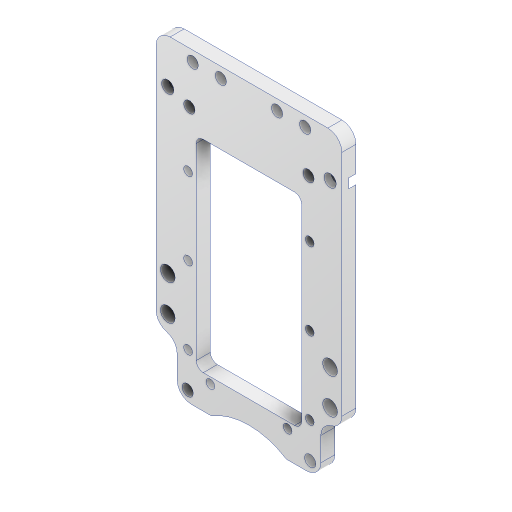
# Autodesk Inventor part: 조인트4고정부
Saved by Autodesk Inventor 2023.2 (Build 272271000, 271)
## iProperties
Created: 2022-01-25
Part Number: 조인트4고정부
Material: 알루미늄 6061
Document SubType Name: Modeling
Designer: BAEK
Density: 2.7 g/cm^3
Appearance: 알루미늄 - 평지
Mass: 26.6199 g
Surface Area: 76.4867 cm^2
Volume: 9.85924 cm^3
Author: BAEK
Autodesk Inventor part; units mm, degrees
ref_plane "YZ Plane" through (0, 0, 0) normal (1, 0, 0) x (0, 1, 0)
ref_plane "XZ Plane" through (0, 0, 0) normal (0, 1, 0) x (-1, 0, 0)
ref_plane "XY Plane" through (0, 0, 0) normal (0, 0, 1) x (1, 0, 0)
sketch "스케치1" plane through (0, 0, 0) normal (0, 0, 1) x (1, 0, 0)
  arc A0 (16.8326, 2) -> (15.3326, 3.5) centre (15.3326, 2) ccw
  line L0 (16.8326, 2) -> (16.8326, 0.5)
  arc A1 (16.8326, 0.5) -> (19.1826, -1.85) centre (19.1826, 0.5) ccw
  line L1 (19.1826, -1.85) -> (21.1826, -1.85)
  arc A2 (22.1826, -2.85) -> (21.1826, -1.85) centre (21.1826, -2.85) ccw
  line L2 (22.1826, -2.85) -> (22.1826, -45.65)
  arc A3 (21.1826, -46.65) -> (22.1826, -45.65) centre (21.1826, -45.65) ccw
  line L3 (21.1826, -46.65) -> (19.1826, -46.65)
  arc A4 (19.1826, -46.65) -> (16.8326, -49) centre (19.1826, -49) ccw
  line L4 (16.8326, -49) -> (16.8326, -51)
  arc A5 (15.8326, -52) -> (16.8326, -51) centre (15.8326, -51) ccw
  line L5 (15.8326, -52) -> (-0.4674, -52)
  arc A6 (-1.4674, -51) -> (-0.4674, -52) centre (-0.4674, -51) ccw
  line L6 (-1.4674, -51) -> (-1.4674, -49)
  arc A7 (-1.4674, -49) -> (-3.8174, -46.65) centre (-3.8174, -49) ccw
  line L7 (-3.8174, -46.65) -> (-5.8174, -46.65)
  arc A8 (-6.8174, -45.65) -> (-5.8174, -46.65) centre (-5.8174, -45.65) ccw
  line L8 (-6.8174, -45.65) -> (-6.8174, -2.85)
  arc A9 (-5.8174, -1.85) -> (-6.8174, -2.85) centre (-5.8174, -2.85) ccw
  line L9 (-5.8174, -1.85) -> (-3.8174, -1.85)
  arc A10 (-3.8174, -1.85) -> (-1.4674, 0.5) centre (-3.8174, 0.5) ccw
  line L10 (-1.4674, 0.5) -> (-1.4674, 2)
  arc A11 (0.0326, 3.5) -> (-1.4674, 2) centre (0.0326, 2) ccw
  circle A12 centre (24.9826, -27.5) radius 1.25
  circle A13 centre (18.6826, -54.8) radius 1.25
  circle A14 centre (-9.6174, -5.5) radius 1.25
  circle A15 centre (-9.6174, -27.5) radius 1.25
  circle A16 centre (-3.3174, -54.8) radius 1.25
  circle A17 centre (24.9826, -49.5) radius 1.25
  circle A18 centre (-9.6174, -49.5) radius 1.25
  circle A19 centre (24.9826, -5.5) radius 1.25
  line L11 (0.0326, 3.5) -> (0.0326, 0.875)
  spline S0 degree 3 poles (0.0326, 0.875) (0.0326, 0.7776) (0.0314, 0.6798) (0.029, 0.5822) (0.0265, 0.4846) (0.0229, 0.3871) (0.0181, 0.29) (0.0132, 0.1929) (0.0072, 0.0961) (0, 0) knots 0 0 0 0 0.333333 0.333333 0.333333 0.666667 0.666667 0.666667 1 1 1 1
  line L12 (15.3652, 0) -> (0, 0)
  spline S1 degree 3 poles (15.3652, 0) (15.3581, 0.0956) (15.352, 0.1921) (15.3472, 0.289) (15.3424, 0.386) (15.3387, 0.4835) (15.3363, 0.5813) (15.3338, 0.679) (15.3326, 0.7771) (15.3326, 0.875) knots 0.000001 0.000001 0.000001 0.000001 0.333333 0.333333 0.333333 0.666667 0.666667 0.666667 1 1 1 1
  line L13 (15.3326, 0.875) -> (15.3326, 3.5)
  line L14 (15.3326, 3.5) -> (0.0326, 3.5)
  circle A20 centre (7.6826, -9.5) radius 5
  line L15 (28.124, 3.5) -> (28.124, -58.5)
  line L16 (-12.7588, 3.5) -> (-12.7588, -58.5)
  line L17 (-12.7588, -58.5) -> (28.124, -58.5)
  line L18 (-12.7588, 3.5) -> (-12.7588, 4.4)
  line L19 (28.124, 4.4) -> (28.124, 3.5)
  line L20 (-12.7588, 4.4) -> (-12.7588, 10)
  line L21 (-12.7588, 10) -> (28.124, 10)
  line L22 (28.124, 10) -> (28.124, 4.4)
  line L23 (7.6826, -52) -> (7.6826, -53)
  line L24 (-6.8174, -24.25) -> (-7.3174, -24.25)
  line L25 (22.1826, -24.25) -> (22.6826, -24.25)
  line L26 (7.6826, 3.5) -> (7.6826, 4.5)
  line L27 (7.6826, 4.5) -> (-5.3174, 4.5)
  line L28 (-7.3174, 2.5) -> (-7.3174, -51)
  line L29 (-5.3174, -53) -> (20.6826, -53)
  line L30 (22.6826, -51) -> (22.6826, 2.5)
  line L31 (20.6826, 4.5) -> (7.6826, 4.5)
  line L32 (-12.7588, -27.5) -> (28.124, -27.5) construction
  line L33 (-3.3174, -54.8) -> (-3.3174, 10) construction
  line L34 (18.6826, -54.8) -> (18.6826, 10) construction
  line L35 (-3.3174, 10) -> (-3.3174, 6.3)
  line L36 (18.6826, 10) -> (18.6826, 6.3)
  circle A21 centre (-3.3174, 6.3) radius 1.25
  circle A22 centre (18.6826, 6.3) radius 1.25
  arc A23 (-7.3174, -51) -> (-5.3174, -53) centre (-5.3174, -51) ccw
  arc A24 (20.6826, -53) -> (22.6826, -51) centre (20.6826, -51) ccw
  arc A25 (22.6826, 2.5) -> (20.6826, 4.5) centre (20.6826, 2.5) ccw
  arc A26 (-5.3174, 4.5) -> (-7.3174, 2.5) centre (-5.3174, 2.5) ccw
  point P0 (0, 0)
  point P1 (-7.3174, 4.5)
  point P2 (-7.3174, -53)
  point P3 (22.6826, -53)
  point P4 (22.6826, 4.5)
  dimension "d4" = 62
  dimension "d9" = 5.6
  dimension "d10" = 1
  dimension "d11" = 0.5
  dimension "d12" = 0.5
  dimension "d13" = 1
  dimension "d14" = 3.7
  dimension "d15" = 3.7
  dimension "d16" = 68.5
  dimension "d18" = 9.4414
  dimension "d19" = 9.4414
  dimension "d22" = 3.7
  dimension "d23" = 3.7
  dimension "d24" = 2.5
  dimension "d25" = 2.5
  dimension "d32" = 2
  dimension "d138" = 2.5
  dimension "d139" = 2.5
  dimension "d140" = 2.5
  dimension "d141" = 2.5
  dimension "d142" = 2.5
  dimension "d143" = 2.5
  dimension "d144" = 2.5
  dimension "d145" = 2.5
  constraints: 74 end point, 32 point on circle, 27 centre point, 12 point on line, 8 tangent, 6 midpoint, 6 perpendicular, 5 horizontal, 5 vertical, 3 equal radius, 2 coincident, 1 parallel, 4 other
  measures "d4" distance of L16.start L16.end
  measures "d9" distance of L18.end L20.end
  measures "d10" distance of L23.start L23.end
  measures "d11" distance of L24.start L24.end
  measures "d12" distance of L25.start L25.end
  measures "d13" distance of L26.start L26.end
  measures "d14" distance from line of L17 L33.start
  measures "d15" distance from line of L17 L34.start
  measures "d16" distance between parallel lines of L17 L21
  measures "d18" distance from line of L16 L33.start
  measures "d19" distance from line of L15 L34.start
  measures "d22" distance of L33.end L35.end
  measures "d23" distance of L34.end L36.end
  measures "d24" diameter of A21
  measures "d25" diameter of A22
  measures "d32" radius of A23
  measures "d138" diameter of A14
  measures "d139" diameter of A15
  measures "d140" diameter of A18
  measures "d141" diameter of A17
  measures "d142" diameter of A12
  measures "d143" diameter of A19
  measures "d144" diameter of A13
  measures "d145" diameter of A16
extrude "돌출2" add sketch "스케치1" along normal blind 4 contours A22 | A21 | L15 L17 L16 L18 L20 L21 L22 L19
sketch "스케치4" plane through (0, 0, 4) normal (0, 0, 1) x (1, 0, 0)
  circle A0 centre (7.6826, -9.5) radius 5
  point P0 (0, 0)
  constraints: 1 centre point
sketch "스케치7" plane through (0, 0, 4) normal (0, 0, 1) x (1, 0, 0)
  line L0 (28.124, 10) -> (-12.7588, 10) projected
  line L1 (-12.7588, 10) -> (28.124, 10)
  line L2 (28.124, 10) -> (28.124, 14)
  line L3 (28.124, 14) -> (-12.7588, 14)
  line L4 (-12.7588, 14) -> (-12.7588, 10)
  line L5 (-12.7588, -58.5) -> (28.124, -58.5) projected
  line L6 (-12.7588, -58.5) -> (28.124, -58.5)
  line L7 (28.124, -58.5) -> (28.124, -62.5)
  line L8 (28.124, -62.5) -> (-12.7588, -62.5)
  line L9 (-12.7588, -62.5) -> (-12.7588, -58.5)
  point P0 (0, 0)
  dimension "d50" = 4
  dimension "d51" = 4
  constraints: 16 end point, 5 perpendicular, 2 horizontal, 1 collinear, 1 point on line
  measures "d50" distance of L0.start L2.end
  measures "d51" distance of L5.end L7.end
extrude "돌출4" add sketch "스케치7" against normal up to surface (4 mm away)
sketch "스케치5" plane through (0, 0, 4) normal (0, 0, 1) x (1, 0, 0)
  line L0 (-12.7588, 14) -> (-12.7588, -62.5) projected
  line L1 (28.124, -62.5) -> (28.124, 14) projected
  circle A0 centre (24.9826, -5.5) radius 1.25 projected
  circle A1 centre (-9.6174, -5.5) radius 1.25 projected
  circle A2 centre (-9.6174, -27.5) radius 1.25 projected
  line L2 (-5.3174, 4.5) -> (20.6826, 4.5) projected
  arc A3 (22.6826, 2.5) -> (20.6826, 4.5) centre (20.6826, 2.5) ccw projected
  line L3 (22.6826, 2.5) -> (22.6826, -51) projected
  arc A4 (20.6826, -53) -> (22.6826, -51) centre (20.6826, -51) ccw projected
  line L4 (20.6826, -53) -> (-5.3174, -53) projected
  arc A5 (-7.3174, -51) -> (-5.3174, -53) centre (-5.3174, -51) ccw projected
  line L5 (-7.3174, -51) -> (-7.3174, 2.5) projected
  arc A6 (-5.3174, 4.5) -> (-7.3174, 2.5) centre (-5.3174, 2.5) ccw projected
  circle A7 centre (-9.6174, -49.5) radius 1.25 projected
  circle A8 centre (-3.3174, -54.8) radius 1.25 projected
  circle A9 centre (24.9826, -49.5) radius 1.25 projected
  circle A10 centre (18.6826, -54.8) radius 1.25 projected
  circle A11 centre (24.9826, -27.5) radius 1.25 projected
  circle A12 centre (-9.7588, -59.5) radius 1.6
  circle A13 centre (25.124, -59.5) radius 1.6
  circle A14 centre (-9.2588, 10.5) radius 1.6
  circle A15 centre (24.624, 10.5) radius 1.6
  line L6 (-12.7588, -62.5) -> (28.124, -62.5) projected
  line L7 (28.124, 14) -> (-12.7588, 14) projected
  point P0 (0, 0)
  dimension "d36" = 3.2
  dimension "d37" = 3.2
  dimension "d38" = 3.2
  dimension "d39" = 3.2
  dimension "d40" = 3
  dimension "d42" = 3.5
  dimension "d44" = 3.5
  dimension "d46" = 3
  dimension "d54" = 3
  dimension "d55" = 3
  dimension "d56" = 3.5
  dimension "d57" = 3.5
  constraints: 4 centre point
  measures "d36" diameter of A12
  measures "d37" diameter of A13
  measures "d38" diameter of A14
  measures "d39" diameter of A15
  measures "d40" distance from line of L0 A12.centre
  measures "d42" distance from line of L0 A14.centre
  measures "d44" distance from line of L1 A15.centre
  measures "d46" distance from line of L1 A13.centre
  measures "d54" distance from line of L6 A12.centre
  measures "d55" distance from line of L6 A13.centre
  measures "d56" distance from line of L7 A14.centre
  measures "d57" distance from line of L7 A15.centre
extrude "돌출3" cut sketch "스케치5" against normal blind 4 contours A12 | A13 | A14 | A15
sketch "스케치8" plane through (0, 0, 4) normal (0, 0, 1) x (1, 0, 0)
  line L0 (-12.7588, 14) -> (28.124, 14) projected
  line L1 (7.6826, 14) -> (7.6826, -136) construction
  circle A0 centre (7.6826, -79.433) radius 20
  line L2 (-12.7588, -62.5) -> (28.124, -62.5) projected
  point P0 (0, 0)
  point P1 (-10.7588, 14)
  point P2 (26.124, 14)
  point P3 (-10.7588, -62.5)
  point P4 (26.124, -62.5)
  point P5 (-2.9604, -62.5)
  point P6 (18.3256, -62.5)
  dimension "d59" = 150
  dimension "d60" = 40
  dimension "d61" = 16.933
  constraints: 2 end point, 1 centre point, 1 midpoint, 1 point on line, 1 vertical
  measures "d59" distance of L1.start L1.end
  measures "d60" diameter of A0
  measures "d61" distance from line of L2 A0.centre
extrude "돌출5" cut sketch "스케치8" against normal up to surface (4 mm away) contours L2 A0 picked at (9.885, -61.852)
sketch "스케치12" plane through (0, 0, 4) normal (0, 0, 1) x (1, 0, 0)
  circle A0 centre (-9.6174, -27.5) radius 1.25 projected
  line L0 (-9.6174, -27.5) -> (-9.6174, -33.6) construction
  line L1 (-9.6174, -33.6) -> (-15.4174, -33.6) construction
  circle A1 centre (-15.4174, -33.6) radius 2.1
  line L2 (-12.7588, 14) -> (-12.7588, -62.5) projected
  line L3 (-15.4174, -33.6) -> (-15.4174, -43.6) construction
  circle A2 centre (-15.4174, -43.6) radius 2.1
  arc A3 (18.3256, -62.5) -> (-2.9604, -62.5) centre (7.6826, -79.433) ccw projected
  line L4 (-15.4174, -33.6) -> (-15.4174, 12.4) construction
  circle A4 centre (-15.4174, 12.4) radius 1.75
  line L5 (28.124, 14) -> (-12.7588, 14) projected
  line L6 (7.6826, 14) -> (7.6826, -59.433) construction
  arc A5 (18.3256, -62.5) -> (-2.9604, -62.5) centre (7.6826, -79.433) ccw projected
  circle A6 centre (30.7826, -33.6) radius 2.1
  line L7 (30.7826, -33.6) -> (30.7826, -43.6) construction
  circle A7 centre (30.7826, -43.6) radius 2.1
  line L8 (30.7826, -33.6) -> (30.7826, 12.4) construction
  circle A8 centre (30.7826, 12.4) radius 1.75
  line L9 (-12.7588, 14) -> (-12.7588, -62.5) projected
  line L10 (-12.7588, 14) -> (-12.7588, 17)
  line L11 (-12.7588, 17) -> (28.124, 17)
  line L12 (28.124, 17) -> (28.124, 14)
  line L13 (28.124, 17) -> (34.124, 17)
  line L14 (34.124, 17) -> (34.124, -48)
  line L15 (34.124, -48) -> (28.124, -48)
  line L16 (28.124, -62.5) -> (28.124, 14) projected
  line L17 (-12.7588, 17) -> (-18.7588, 17)
  line L18 (-18.7588, 17) -> (-18.7588, -48)
  line L19 (-18.7588, -48) -> (-12.7588, -48)
  point P0 (0, 0)
  point P1 (-12.7588, -60.5)
  point P2 (28.124, -60.5)
  dimension "d83" = 6.1
  dimension "d84" = 5.8
  dimension "d85" = 4.2
  dimension "d87" = 10
  dimension "d88" = 4.2
  dimension "d89" = 46
  dimension "d90" = 3
  dimension "d91" = 6
  dimension "d92" = 65
  dimension "d93" = 6
  dimension "d128" = 3.5
  constraints: 32 end point, 6 centre point, 6 coincident, 6 symmetric about line, 6 vertical, 5 perpendicular, 3 point on line, 2 point on circle, 1 midpoint, 1 parallel, 3 other
  measures "d83" distance of L0.start L0.end
  measures "d84" distance of L0.end L1.end
  measures "d85" diameter of A1
  measures "d87" distance of L3.start L3.end
  measures "d88" diameter of A2
  measures "d89" distance of L3.start L4.end
  measures "d90" distance of L2.start L10.end
  measures "d91" distance of L11.end L13.end
  measures "d92" distance of L13.end L14.end
  measures "d93" distance of L10.end L17.end
  measures "d128" diameter of A4
extrude "돌출8" add sketch "스케치12" against normal blind 4 contours L10 L11 L12 L5 | L2 L19 L18 L17 L10 | L12 L13 L14 L15 L16
sketch "스케치13" plane through (0, 0, 4) normal (0, 0, 1) x (1, 0, 0)
  circle A0 centre (-15.4174, 12.4) radius 1.75 projected
  circle A1 centre (-15.4174, -43.6) radius 2.1 projected
  circle A2 centre (-15.4174, -33.6) radius 2.1 projected
  circle A3 centre (30.7826, 12.4) radius 1.75 projected
  circle A4 centre (30.7826, -43.6) radius 2.1 projected
  circle A5 centre (30.7826, -33.6) radius 2.1 projected
  circle A6 centre (24.9826, -27.5) radius 1.25 projected
  circle A7 centre (18.6826, -54.8) radius 1.25 projected
  circle A8 centre (24.9826, -49.5) radius 1.25 projected
  circle A9 centre (-3.3174, -54.8) radius 1.25 projected
  circle A10 centre (-9.6174, -49.5) radius 1.25 projected
  arc A11 (20.6826, -53) -> (22.6826, -51) centre (20.6826, -51) ccw projected
  line L0 (20.6826, -53) -> (-5.3174, -53) projected
  arc A12 (-7.3174, -51) -> (-5.3174, -53) centre (-5.3174, -51) ccw projected
  line L1 (-7.3174, -51) -> (-7.3174, 2.5) projected
  arc A13 (-5.3174, 4.5) -> (-7.3174, 2.5) centre (-5.3174, 2.5) ccw projected
  line L2 (-5.3174, 4.5) -> (20.6826, 4.5) projected
  arc A14 (22.6826, 2.5) -> (20.6826, 4.5) centre (20.6826, 2.5) ccw projected
  line L3 (22.6826, 2.5) -> (22.6826, -51) projected
  circle A15 centre (-9.6174, -27.5) radius 1.25 projected
  circle A16 centre (-9.6174, -5.5) radius 1.25 projected
  circle A17 centre (24.9826, -5.5) radius 1.25 projected
  arc A18 (18.3256, -62.5) -> (-2.9604, -62.5) centre (7.6826, -79.433) ccw projected
  line L4 (18.3256, -62.5) -> (28.124, -62.5) projected
  line L5 (28.124, -62.5) -> (28.124, -48) projected
  line L6 (28.124, -48) -> (34.124, -48) projected
  line L7 (34.124, -48) -> (34.124, 17) projected
  line L8 (34.124, 17) -> (-18.7588, 17) projected
  line L9 (-18.7588, 17) -> (-18.7588, -48) projected
  line L10 (-18.7588, -48) -> (-12.7588, -48) projected
  line L11 (-12.7588, -48) -> (-12.7588, -62.5) projected
  line L12 (-12.7588, -62.5) -> (-2.9604, -62.5) projected
  circle A19 centre (-9.7588, -59.5) radius 1.6 projected
  circle A20 centre (-9.2588, 10.5) radius 1.6 projected
  circle A21 centre (25.124, -59.5) radius 1.6 projected
  circle A22 centre (24.624, 10.5) radius 1.6 projected
  line L13 (-18.7588, 17) -> (34.124, 17) projected
  line L14 (-18.7588, 17) -> (-18.7588, 25)
  line L15 (34.124, 17) -> (34.124, -48) projected
  line L16 (34.124, 17) -> (34.124, 25)
  line L17 (34.124, 25) -> (-18.7588, 25)
  point P0 (0, 0)
  dimension "d97" = 8
  dimension "d98" = 8
  constraints: 6 end point, 2 vertical
  measures "d97" distance of L8.end L14.end
  measures "d98" distance of L7.end L16.end
extrude "돌출9" add sketch "스케치13" against normal blind 4 contours L8 L14 L17 L16
sketch "스케치14" plane through (0, 0, 4) normal (0, 0, 1) x (1, 0, 0)
  circle A0 centre (-15.4174, 12.4) radius 1.75 projected
  circle A1 centre (-15.4174, -43.6) radius 2.1 projected
  circle A2 centre (-15.4174, -33.6) radius 2.1 projected
  circle A3 centre (30.7826, 12.4) radius 1.75 projected
  circle A4 centre (30.7826, -43.6) radius 2.1 projected
  circle A5 centre (30.7826, -33.6) radius 2.1 projected
  circle A6 centre (24.9826, -27.5) radius 1.25 projected
  circle A7 centre (18.6826, -54.8) radius 1.25 projected
  circle A8 centre (24.9826, -49.5) radius 1.25 projected
  circle A9 centre (-3.3174, -54.8) radius 1.25 projected
  circle A10 centre (-9.6174, -49.5) radius 1.25 projected
  arc A11 (20.6826, -53) -> (22.6826, -51) centre (20.6826, -51) ccw projected
  line L0 (20.6826, -53) -> (-5.3174, -53) projected
  arc A12 (-7.3174, -51) -> (-5.3174, -53) centre (-5.3174, -51) ccw projected
  line L1 (-7.3174, -51) -> (-7.3174, 2.5) projected
  arc A13 (-5.3174, 4.5) -> (-7.3174, 2.5) centre (-5.3174, 2.5) ccw projected
  line L2 (-5.3174, 4.5) -> (20.6826, 4.5) projected
  arc A14 (22.6826, 2.5) -> (20.6826, 4.5) centre (20.6826, 2.5) ccw projected
  line L3 (22.6826, 2.5) -> (22.6826, -51) projected
  circle A15 centre (-9.6174, -27.5) radius 1.25 projected
  circle A16 centre (-9.6174, -5.5) radius 1.25 projected
  circle A17 centre (24.9826, -5.5) radius 1.25 projected
  arc A18 (18.3256, -62.5) -> (-2.9604, -62.5) centre (7.6826, -79.433) ccw projected
  line L4 (18.3256, -62.5) -> (28.124, -62.5) projected
  line L5 (28.124, -62.5) -> (28.124, -48) projected
  line L6 (28.124, -48) -> (34.124, -48) projected
  line L7 (34.124, -48) -> (34.124, 25) projected
  line L8 (34.124, 25) -> (-18.7588, 25) projected
  line L9 (-18.7588, 25) -> (-18.7588, -48) projected
  line L10 (-18.7588, -48) -> (-12.7588, -48) projected
  line L11 (-12.7588, -48) -> (-12.7588, -62.5) projected
  line L12 (-12.7588, -62.5) -> (-2.9604, -62.5) projected
  circle A19 centre (-9.7588, -59.5) radius 1.6 projected
  circle A20 centre (-9.2588, 10.5) radius 1.6 projected
  circle A21 centre (25.124, -59.5) radius 1.6 projected
  circle A22 centre (24.624, 10.5) radius 1.6 projected
  line L13 (-18.7588, 25) -> (34.124, 25) projected
  line L14 (7.6826, 25) -> (7.6826, 19) construction
  line L15 (-18.7588, -48) -> (-18.7588, 25) projected
  line L16 (-18.7588, 22) -> (34.124, 22) construction
  line L17 (34.124, 25) -> (34.124, -48) projected
  circle A23 centre (23.6826, 22) radius 1.6
  circle A24 centre (-0.3174, 22) radius 1.6
  circle A25 centre (-8.3174, 22) radius 1.6
  circle A26 centre (15.6826, 22) radius 1.6
  point P0 (0, 0)
  dimension "d101" = 6
  dimension "d103" = 3.2
  dimension "d104" = 3.2
  dimension "d105" = 3.2
  dimension "d106" = 3.2
  dimension "d107" = 8
  dimension "d108" = 8
  dimension "d109" = 8
  dimension "d110" = 8
  constraints: 6 point on line, 4 centre point, 4 end point, 1 midpoint, 1 perpendicular, 1 vertical
  measures "d101" distance of L14.start L14.end
  measures "d103" diameter of A23
  measures "d104" diameter of A24
  measures "d105" diameter of A25
  measures "d106" diameter of A26
  measures "d107" distance of A23.centre A26.centre
  measures "d108" distance of A25.centre A24.centre
  measures "d109" distance from line of L14 A24.centre
  measures "d110" distance from line of L14 A26.centre
extrude "돌출10" cut sketch "스케치14" against normal up to surface (4 mm away) contours A23 | A24 | A25 | A26
fillet "모깎기7" radius 4 8 edges at (-18.7588, 25, 2) (34.124, 25, 2) (34.124, -48, 2) (28.124, -48, 2) (-12.7588, -48, 2) (-18.7588, -48, 2) (-12.7588, -62.5, 2) (28.124, -62.5, 2)
sketch "스케치18" plane through (0, 0, 0) normal (0, 0, -1) x (-1, 0, 0)
  arc A0 (-28.124, -58.5) -> (-24.124, -62.5) centre (-24.124, -58.5) ccw projected
  line L0 (-24.124, -62.5) -> (-18.3256, -62.5) projected
  arc A1 (2.9604, -62.5) -> (-18.3256, -62.5) centre (-7.6826, -79.433) ccw projected
  line L1 (2.9604, -62.5) -> (8.7588, -62.5) projected
  arc A2 (8.7588, -62.5) -> (12.7588, -58.5) centre (8.7588, -58.5) ccw projected
  line L2 (12.7588, -52) -> (12.7588, -58.5) projected
  arc A3 (15.7588, -48.127) -> (12.7588, -52) centre (16.7588, -52) ccw projected
  arc A4 (15.7588, -48.127) -> (18.7588, -44.254) centre (14.7588, -44.254) ccw projected
  line L3 (18.7588, -44.254) -> (18.7588, 21) projected
  arc A5 (18.7588, 21) -> (14.7588, 25) centre (14.7588, 21) ccw projected
  line L4 (14.7588, 25) -> (-30.124, 25) projected
  arc A6 (-30.124, 25) -> (-34.124, 21) centre (-30.124, 21) ccw projected
  line L5 (-34.124, 21) -> (-34.124, -44) projected
  arc A7 (-34.124, -44) -> (-31.124, -47.873) centre (-30.124, -44) ccw projected
  arc A8 (-28.124, -51.746) -> (-31.124, -47.873) centre (-32.124, -51.746) ccw projected
  line L6 (-28.124, -51.746) -> (-28.124, -58.5) projected
  circle A9 centre (-15.6826, 22) radius 1.6 projected
  circle A10 centre (8.3174, 22) radius 1.6 projected
  circle A11 centre (-23.6826, 22) radius 1.6 projected
  circle A12 centre (0.3174, 22) radius 1.6 projected
  circle A13 centre (15.4174, 12.4) radius 1.75 projected
  circle A14 centre (15.4174, -43.6) radius 2.1 projected
  circle A15 centre (15.4174, -33.6) radius 2.1 projected
  circle A16 centre (-30.7826, 12.4) radius 1.75 projected
  circle A17 centre (-30.7826, -43.6) radius 2.1 projected
  circle A18 centre (-30.7826, -33.6) radius 2.1 projected
  circle A19 centre (-24.9826, -27.5) radius 1.25 projected
  circle A20 centre (-18.6826, -54.8) radius 1.25 projected
  circle A21 centre (-24.9826, -49.5) radius 1.25 projected
  circle A22 centre (3.3174, -54.8) radius 1.25 projected
  circle A23 centre (9.6174, -49.5) radius 1.25 projected
  arc A24 (-22.6826, -51) -> (-20.6826, -53) centre (-20.6826, -51) ccw projected
  line L7 (-22.6826, 2.5) -> (-22.6826, -51) projected
  arc A25 (-20.6826, 4.5) -> (-22.6826, 2.5) centre (-20.6826, 2.5) ccw projected
  line L8 (5.3174, 4.5) -> (-20.6826, 4.5) projected
  arc A26 (7.3174, 2.5) -> (5.3174, 4.5) centre (5.3174, 2.5) ccw projected
  line L9 (7.3174, -51) -> (7.3174, 2.5) projected
  arc A27 (5.3174, -53) -> (7.3174, -51) centre (5.3174, -51) ccw projected
  line L10 (-20.6826, -53) -> (5.3174, -53) projected
  circle A28 centre (9.6174, -27.5) radius 1.25 projected
  circle A29 centre (9.6174, -5.5) radius 1.25 projected
  circle A30 centre (-24.9826, -5.5) radius 1.25 projected
  circle A31 centre (9.7588, -59.5) radius 1.6 projected
  circle A32 centre (9.2588, 10.5) radius 1.6 projected
  circle A33 centre (-25.124, -59.5) radius 1.6 projected
  circle A34 centre (-24.624, 10.5) radius 1.6 projected
  circle A35 centre (-30.7826, 12.4) radius 3.6
  circle A36 centre (15.4174, 12.4) radius 3.6
  point P0 (0, 0)
  dimension "d134" = 7.2
  dimension "d135" = 7.2
  constraints: 2 centre point, 2 coincident
  measures "d134" diameter of A35
  measures "d135" diameter of A36
extrude "돌출12" cut sketch "스케치18" against normal blind 2 contours A35 L5 | L5 A35 | A36 L3 | L3 A36
equation "\"d111\" = d104"
